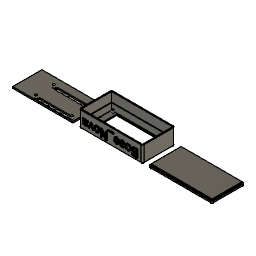
MYPOD (Autodesk Fusion 360 design; units mm, degrees)
part number: 2026-06-26-11-47-34-600
Autodesk Fusion 360 part; units mm, degrees
note: some values were not read from the file. Chosen so that the rebuilt part matches the saved one: which bodies a step acts on; which face or edge a step refers to.
sketch "Sketch9" plane through (0, 0, 0) normal (0, 0, 1) x (1, 0, 0)
  line L0 (-41, 21) -> (41, 21)
  line L1 (41, 21) -> (41, -21)
  line L2 (41, -21) -> (-41, -21)
  line L3 (-41, -21) -> (-41, 21)
  line L4 (-31.3013, 17.7789) -> (32.6988, 17.7789)
  line L5 (32.6988, 17.7789) -> (32.6988, -0.7211)
  line L6 (32.6988, -0.7211) -> (-31.3013, -0.7211)
  line L7 (-31.3013, -0.7211) -> (-31.3013, 17.7789)
  circle A0 centre (-35.3012, 16.9789) radius 1.2042
  circle A1 centre (-35.3552, 0.4127) radius 1.204
  circle A2 centre (-27.9079, -12.5947) radius 6.25
  circle A3 centre (-13.9079, -12.5947) radius 6.25
  circle A4 centre (0.0921, -12.5947) radius 6.25
  circle A5 centre (14.0921, -12.5947) radius 6.25
  circle A6 centre (28.0921, -12.5947) radius 6.25
  dimension "d49" = 82
  dimension "d50" = 42
  dimension "d51" = 41
  dimension "d52" = 21
  dimension "d53" = 2.408
  dimension "d54" = 12.5
  dimension "d55" = 12.5
  dimension "d56" = 12.5
  dimension "d57" = 12.5
  dimension "d58" = 12.5
  constraint horizontal L0
  constraint vertical L1
  constraint horizontal L2
  constraint vertical L3
  constraint horizontal L4
  constraint vertical L5
  constraint horizontal L6
  constraint vertical L7
  measures "d49" distance of L0.start L0.end
  measures "d50" distance of L0.start L2.end
  measures "d51" distance of origin L1
  measures "d52" distance of origin L0
  measures "d53" diameter of A1
  measures "d54" diameter of A2
  measures "d55" diameter of A3
  measures "d56" diameter of A4
  measures "d57" diameter of A5
  measures "d58" diameter of A6
extrude "Extrude16" add sketch "Sketch9" along normal blind 22 contours L0 L1 L2 L3 | L4 L5 L6 L7 | A0 | A1 | A2 | A3 | A4 | A5 | A6 makes body 1
shell "Shell4" thickness 1.5 removed faces 1 at (-13.6667, 7, 22) on bodies 1
extrude "Extrude17" cut sketch "Sketch9" along normal blind 2 contours L4 L5 L6 L7 | A2 | A3 | A4 | A5 | A6 bodies 1
extrude "Extrude18" cut sketch "Sketch9" along normal blind 5 contours A0 | A1 bodies 1
extrude "Extrude19" add sketch "Sketch9" along normal blind 5 contours A0 | A1 bodies 1
sketch "Sketch10" plane through (0, 0, 0) normal (0, 0, 1) x (1, 0, 0)
  line L0 (58, 18) -> (140, 18)
  line L1 (140, 18) -> (140, -24)
  line L2 (140, -24) -> (58, -24)
  line L3 (58, -24) -> (58, 18)
  dimension "d68" = 82
  dimension "d69" = 42
  constraint horizontal L0
  constraint vertical L1
  constraint horizontal L2
  constraint vertical L3
  measures "d68" distance of L0.start L0.end
  measures "d69" distance of L0.start L2.end
extrude "Extrude20" add sketch "Sketch10" along normal blind 2 separate body makes body 2
extrude "Extrude21" add 1 faces at (85.3333, -10, 2) along direction (0, 0, 1) blind 2 on bodies 2 bodies 2
shell "Shell5" thickness 1.5 removed faces 1 at (85.3333, -10, 4) on bodies 2
extrude "Extrude22" add 1 faces at (85.8333, 3.5, 1.5) along direction (0, 0, 1) blind 2 on bodies 2 bodies 2
sketch "Sketch12" plane through (0, 0, 0) normal (0, 0, 1) x (1, 0, 0)
  line L0 (-39.5, 19.5) -> (39.5, 19.5)
  line L1 (39.5, 19.5) -> (39.5, -19.5)
  line L2 (39.5, -19.5) -> (-39.5, -19.5)
  line L3 (-39.5, -19.5) -> (-39.5, 19.5)
  line L4 (-39, -19) -> (39, -19)
  line L5 (39, -19) -> (39, 19)
  line L6 (39, 19) -> (-39, 19)
  line L7 (-39, 19) -> (-39, -19)
  circle A0 centre (-11.5, -16.3) radius 1.5
  circle A1 centre (35, -16.3) radius 1.5
  circle A2 centre (35, 7) radius 1.5
  circle A3 centre (-11.5, 7) radius 1.5
  line L8 (-9, 9) -> (33, 9)
  line L9 (33, 9) -> (33, -18)
  line L10 (33, -18) -> (-9, -18)
  line L11 (-9, -18) -> (-9, 9)
  line L12 (-14, 5) -> (37, 5)
  line L13 (37, 5) -> (37, -14)
  line L14 (37, -14) -> (-14, -14)
  line L15 (-14, -14) -> (-14, 5)
  dimension "d85" = 3
  dimension "d86" = 3
  dimension "d87" = 3
  dimension "d88" = 3
  constraint horizontal L0
  constraint vertical L1
  constraint horizontal L2
  constraint vertical L3
  constraint horizontal L4
  constraint vertical L5
  constraint horizontal L6
  constraint vertical L7
  constraint horizontal L8
  constraint vertical L9
  constraint horizontal L10
  constraint vertical L11
  constraint horizontal L12
  constraint vertical L13
  constraint horizontal L14
  constraint vertical L15
  measures "d85" diameter of A0
  measures "d86" diameter of A1
  measures "d87" diameter of A3
  measures "d88" diameter of A2
extrude "Extrude23" add sketch "Sketch12" along normal blind 10 contours L0 L1 L2 L3 bodies 1
sketch "Sketch13" plane through (0, 0, 0) normal (0, 0, 1) x (1, 0, 0)
extrude "Extrude24" add sketch "Sketch12" along normal blind 2 separate body contours L4 L5 L6 L7 | A0 | A1 | A2 | A3 | L8 L9 L11 L12 | L9 L11 L12 L14 | L11 L12 L14 L15 | L9 L12 L13 L14 | L9 L10 L11 L14 makes body 3
move_body "Move1" bodies 3 to x (1, 0, 0) y (0, 1, 0) z (0, 0, 1) at (0, 0, 10)
extrude "Extrude25" add sketch "Sketch12" along normal blind 3 separate body contours A0 | A1 | A2 | A3 makes body 4 at (36.4981, 6.9252, 2) makes body 5 at (-10.0019, 6.9252, 2) makes body 6 at (35.4063, -14.8561, 2) makes body 7 at (-10.0019, -16.3748, 2)
move_body "Move2" bodies 7 5 6 4 to x (1, 0, 0) y (0, 1, 0) z (0, 0, 1) at (0, 0, 10)
move_body "Move3" bodies 7 6 4 5 to x (1, 0, 0) y (0, 1, 0) z (0, 0, 1) at (0, 0, 2)
extrude "Extrude26" add sketch "Sketch12" along normal blind 2 separate body contours L8 L9 L11 L12 | L9 L10 L11 L14 makes body 8 at (5, 6.3333, 0) makes body 9 at (5, -16.6667, 0)
move_body "Move4" bodies 9 8 to x (1, 0, 0) y (0, 1, 0) z (0, 0, 1) at (0, 0, 10)
extrude "Extrude27" cut 1 faces at (5, 6.3333, 12) along direction (0, 0, -1) blind 2 on bodies 8 bodies 3 8
extrude "Extrude28" cut 1 faces at (5, -16.6667, 12) along direction (0, 0, -1) blind 2 on bodies 9 bodies 3 9
sketch "Sketch14" plane through (0, -21, 0) normal (0, -1, 0) x (1, 0, 0)
  line L0 (-41, 0) -> (41, 0)
  line L1 (41, 0) -> (41, 22)
  line L2 (41, 22) -> (-41, 22)
  line L3 (-41, 22) -> (-41, 0)
  line L4 (35, 20) -> (-35, 20) construction
  line L5 (-35, 20) -> (-35, 5) construction
  line L6 (-35, 5) -> (35, 5) construction
  line L7 (35, 5) -> (35, 20) construction
  dimension "d97" = 10
  text T0 "Bose_Nova" font "Arial" height 10 align left top in box 70 x 15 at (35, 20) x (-1, 0) y (0, -1) spacing 1
extrude "Extrude29" add sketch "Sketch14" along normal blind 1 text T0 bodies 2 1 3 4 5 6 7
sketch "Sketch15" plane through (0, 0, 0) normal (0, 0, 1) x (1, 0, 0)
fillet "Fillet1" radius 2 1 edges at (0, -21, 0) on bodies 1
fillet "Fillet2" radius 2 3 edges at (-41, -21, 12) (-41, -20.4142, 0.5858) (-41, 1, 0) on bodies 1
fillet "Fillet3" radius 2 3 edges at (41, 1, 0) (41, -20.4142, 0.5858) (41, -21, 12) on bodies 1
fillet "Fillet4" radius 2 5 edges at (-41, 21, 12) (-40.4142, 21, 0.5858) (0, 21, 0) (40.4142, 21, 0.5858) (41, 21, 12) on bodies 1
sketch "Sketch16" plane through (0, 21, 0) normal (0, 1, 0) x (-1, 0, 0)
  line L0 (39, 2) -> (39, 22)
  line L1 (39, 22) -> (-39, 22)
  line L2 (-39, 22) -> (-39, 2)
  line L3 (-39, 2) -> (39, 2)
  line L4 (23.6693, 18.6941) -> (-19.4753, 19.3868) construction
  line L5 (-19.4753, 19.3868) -> (-19.6693, 7.3059) construction
  line L6 (-19.6693, 7.3059) -> (23.4753, 6.6132) construction
  line L7 (23.4753, 6.6132) -> (23.6693, 18.6941) construction
  dimension "d109" = 10
  text T0 "My_Pod" font "Arial" height 10 align left top in box 43.1502 x 12.0824 at (23.6693, 18.6941) x (-0.999871, 0.016055) y (-0.016055, -0.999871) spacing 1
extrude "Extrude30" add sketch "Sketch16" along normal blind 1.5 text T0 bodies 1
fillet "Fillet5" radius 2 1 edges at (99, 18, 0) on bodies 2
fillet "Fillet6" radius 2 1 edges at (99, -24, 0) on bodies 2
fillet "Fillet7" radius 2 5 edges at (58, -24, 3) (58, -23.4142, 0.5858) (58, -3, 0) (58, 17.4142, 0.5858) (58, 18, 3) on bodies 2
fillet "Fillet8" radius 2 5 edges at (140, 18, 3) (140, 17.4142, 0.5858) (140, -3, 0) (140, -23.4142, 0.5858) (140, -24, 3) on bodies 2
extrude "Extrude31" add 1 faces at (85.8333, 3.5, 3.5) along direction (0, 0, 1) blind 2 on bodies 2 bodies 2
sketch "Sketch17" plane through (0, 0, 0) normal (0, 0, 1) x (1, 0, 0)
sketch "Sketch18" plane through (0, -24, 0) normal (0, -1, 0) x (1, 0, 0)
  line L0 (138, 2) -> (138, 4)
  line L1 (138, 4) -> (60, 4)
  line L2 (60, 4) -> (60, 2)
  line L3 (60, 2) -> (138, 2)
move_body "Move5" bodies 2 to x (1, 0, 0) y (0, 1, 0) z (0, 0, 1) at (-99, 0, 25)
move_body "Move6" bodies 2 to x (1, 0, 0) y (0, 1, 0) z (0, 0, 1) at (0, 3, 0)
sketch "Sketch19" plane through (0, -21, 0) normal (0, -1, 0) x (1, 0, 0)
  line L0 (39, 27) -> (39, 29)
  line L1 (39, 29) -> (-39, 29)
  line L2 (-39, 29) -> (-39, 27)
  line L3 (-39, 27) -> (39, 27)
move_body "Move7" bodies 2 to x (-1, 0, 0) y (0, 1, 0) z (0, 0, -1) at (-78, 0, 54)
move_body "Move8" bodies 2 to x (1, 0, 0) y (0, 1, 0) z (0, 0, 1) at (78, 0, 0)
move_body "Move9" bodies 2 to x (1, 0, 0) y (0, 1, 0) z (0, 0, 1) at (0, 0, -3)
move_body "Move10" bodies 2 to x (1, 0, 0) y (0, 1, 0) z (0, 0, 1) at (0, 0, 30)
move_body "Move11" bodies 4 3 6 5 7 to x (1, 0, 0) y (0, 1, 0) z (0, 0, 1) at (0, 0, 20)
move_body "Move12" bodies 2 to x (1, 0, 0) y (0, 1, 0) z (0, 0, 1) at (0, 0, 10)
move_body "Move13" bodies 2 to x (-1, 0, 0) y (0, 1, 0) z (0, 0, -1) at (90, 0, 74)
move_body "Move14" bodies 2 to x (1, 0, 0) y (0, 1, 0) z (0, 0, 1) at (0, 0, -8)
move_body "Move15" bodies 4 3 5 7 6 to x (1, 0, 0) y (0, 1, 0) z (0, 0, 1) at (-90, 0, -30)
equation "d98 = 'Bose_Nova'"
equation "d110 = 'My_Pod'"
